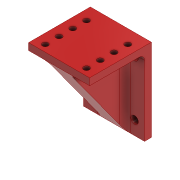
# Autodesk Inventor part: support
Saved by Autodesk Inventor 2020 (Build 240168000, 168)
## iProperties
Created: 2019-12-23
Part Number: support
Material: Generic
Document SubType Name: Modeling
Designer: ball
Density: 1 g/cm^3
Appearance: Default
Author: ball
Autodesk Inventor part; units mm, degrees
ref_plane "Work Plane1" through (172, 48, 15.3) normal (0, -1, 0) x (-1, 0, 0)
sketch "Sketch1" plane through (172, 48, 15.3) normal (0, -1, 0) x (-1, 0, 0)
  circle A0 centre (12, -16.7) radius 1.7 construction
  circle A1 centre (12, -32.7) radius 1.7 construction
  circle A2 centre (-12, 7.3) radius 1.7 construction
  circle A3 centre (-12, 15.3) radius 1.7 construction
  circle A4 centre (-12, 23.3) radius 1.7 construction
  circle A5 centre (-12, -24.7) radius 1.7 construction
  circle A6 centre (12, 23.3) radius 1.7 construction
  circle A7 centre (12, -56.7) radius 1.7 construction
  circle A8 centre (12, -48.7) radius 1.7 construction
  circle A9 centre (12, -40.7) radius 1.7 construction
  circle A10 centre (12, -8.7) radius 1.7 construction
  circle A11 centre (-12, -16.7) radius 1.7 construction
  circle A12 centre (12, -24.7) radius 1.7 construction
  circle A13 centre (-12, -0.7) radius 1.7 construction
  circle A14 centre (-12, -40.7) radius 1.7 construction
  circle A15 centre (-12, -48.7) radius 1.7 construction
  circle A16 centre (-12, -56.7) radius 1.7 construction
  circle A17 centre (-12, -32.7) radius 1.7 construction
  circle A18 centre (12, -80.7) radius 1.7 construction
  circle A19 centre (12, 15.3) radius 1.7 construction
  circle A20 centre (12, 7.3) radius 1.7 construction
  circle A21 centre (12, -0.7) radius 1.7 construction
  circle A22 centre (-12, -8.7) radius 1.7 construction
  circle A23 centre (-12, -80.7) radius 1.7 construction
  line L0 (10.05, 51.5627) -> (14.45, 51.5627) construction
  line L1 (14.45, 51.5627) -> (14.45, 45.5871) construction
  line L2 (14.45, 45.5871) -> (10.05, 45.5871) construction
  line L3 (10.05, 45.5871) -> (10.05, 51.5627) construction
  line L4 (10.05, -66.0122) -> (14.45, -66.0122) construction
  line L5 (14.45, -66.0122) -> (14.45, -71.9878) construction
  line L6 (14.45, -71.9878) -> (10.05, -71.9878) construction
  line L7 (10.05, -71.9878) -> (10.05, -66.0122) construction
  line L8 (-10.05, 75.3622) -> (-14.45, 75.3622) construction
  line L9 (-14.45, 75.3622) -> (-14.45, 81.3378) construction
  line L10 (-14.45, 81.3378) -> (-10.05, 81.3378) construction
  line L11 (-10.05, 81.3378) -> (-10.05, 75.3622) construction
  line L12 (-14.45, 56.302) -> (-10.05, 56.302) construction
  line L13 (-10.05, 56.302) -> (-10.05, 50.3264) construction
  line L14 (-10.05, 50.3264) -> (-14.45, 50.3264) construction
  line L15 (-14.45, 50.3264) -> (-14.45, 56.302) construction
  line L16 (9.5604, 33.925) -> (12.375, 35.55) construction
  line L17 (12.375, 35.55) -> (15.1896, 33.925) construction
  line L18 (15.1896, 33.925) -> (15.1896, 30.675) construction
  line L19 (15.1896, 30.675) -> (12.375, 29.05) construction
  line L20 (12.375, 29.05) -> (9.5604, 30.675) construction
  line L21 (9.5604, 30.675) -> (9.5604, 33.925) construction
  line L22 (2.8106, 33.925) -> (5.6252, 35.55) construction
  line L23 (5.6252, 35.55) -> (8.4398, 33.925) construction
  line L24 (8.4398, 33.925) -> (8.4398, 30.675) construction
  line L25 (8.4398, 30.675) -> (5.6252, 29.05) construction
  line L26 (5.6252, 29.05) -> (2.8106, 30.675) construction
  line L27 (2.8106, 30.675) -> (2.8106, 33.925) construction
  line L28 (3.2502, 68.3) -> (3.2502, 81) construction
  line L29 (3.2502, 81) -> (8.0002, 81) construction
  line L30 (8.0002, 81) -> (8.0002, 68.3) construction
  line L31 (8.0002, 68.3) -> (3.2502, 68.3) construction
  circle A24 centre (12.375, 40.3) radius 1.7 construction
  circle A25 centre (5.6252, 40.3) radius 1.7 construction
  line L32 (10.0002, 81) -> (14.75, 81) construction
  line L33 (14.75, 81) -> (14.75, 68.3) construction
  line L34 (14.75, 68.3) -> (10.0002, 68.3) construction
  line L35 (10.0002, 68.3) -> (10.0002, 81) construction
  line L36 (3.2502, 53.6) -> (3.2502, 66.3) construction
  line L37 (3.2502, 66.3) -> (8.0002, 66.3) construction
  line L38 (8.0002, 66.3) -> (8.0002, 53.6) construction
  line L39 (8.0002, 53.6) -> (3.2502, 53.6) construction
  circle A26 centre (-7.75, 60) radius 1.7 construction
  circle A27 centre (-7.75, -75) radius 1.7 construction
  line L40 (-6.125, 72.8146) -> (-4.5, 70) construction
  line L41 (-4.5, 70) -> (-6.125, 67.1854) construction
  line L42 (-6.125, 67.1854) -> (-9.375, 67.1854) construction
  line L43 (-9.375, 67.1854) -> (-11, 70) construction
  line L44 (-11, 70) -> (-9.375, 72.8146) construction
  line L45 (-9.375, 72.8146) -> (-6.125, 72.8146) construction
  line L46 (-6.125, -62.1854) -> (-4.5, -65) construction
  line L47 (-4.5, -65) -> (-6.125, -67.8146) construction
  line L48 (-6.125, -67.8146) -> (-9.375, -67.8146) construction
  line L49 (-9.375, -67.8146) -> (-11, -65) construction
  line L50 (-11, -65) -> (-9.375, -62.1854) construction
  line L51 (-9.375, -62.1854) -> (-6.125, -62.1854) construction
  line L52 (17.75, 85) -> (-17.75, 85) construction
  line L53 (-17.75, 85) -> (-17.75, -85) construction
  line L54 (-17.75, -85) -> (17.75, -85) construction
  line L55 (17.75, -85) -> (17.75, 85) construction
  line L56 (172, 15.3) -> (-20, 15.3) construction
  line L57 (-17.75, 15.3) -> (17.75, 15.3)
  line L58 (17.75, 15.3) -> (17.75, -20.6375)
  line L59 (17.75, -20.6375) -> (-17.75, -20.6375)
  line L60 (-17.75, 15.3) -> (-17.75, -20.6375)
  circle A28 centre (-12, 7.3) radius 1.7
  circle A29 centre (-12, -0.7) radius 1.7
  circle A30 centre (-12, -8.7) radius 1.7
  circle A31 centre (-12, -16.7) radius 1.7
  circle A32 centre (12, -16.7) radius 1.7
  circle A33 centre (12, -8.7) radius 1.7
  circle A34 centre (12, -0.7) radius 1.7
  circle A35 centre (12, 7.3) radius 1.7
  constraints: 8 centre point, 8 coincident, 8 concentric, 8 end point, 6 point on line, 2 perpendicular
extrude "Extrusion1" add sketch "Sketch1" along normal blind 4
ref_plane "Work Plane2" through (0, 0, 0) normal (0, 0, 1) x (1, 0, 0)
sketch "Sketch2" plane through (0, 0, 0) normal (0, 0, 1) x (1, 0, 0)
  line L0 (192, 0) -> (192, 48) construction
  line L1 (0, 48) -> (192, 48) construction
  line L2 (0, 0) -> (0, 48) construction
  line L3 (0, 0) -> (192, 0) construction
  circle A0 centre (168, 24) radius 7 construction
  circle A1 centre (144, 24) radius 7 construction
  arc A2 (160.9289, 33.8995) -> (158.1005, 31.0711) centre (159.5147, 32.4853) ccw construction
  line L4 (161.4142, 33.4142) -> (160.9289, 33.8995) construction
  arc A3 (158.5858, 30.5858) -> (161.4142, 33.4142) centre (160, 32) ccw construction
  line L5 (158.1005, 31.0711) -> (158.5858, 30.5858) construction
  line L6 (156.6863, 26) -> (155.3137, 26) construction
  arc A4 (156.6863, 22) -> (156.6863, 26) centre (156.6863, 24) ccw construction
  line L7 (155.3137, 22) -> (156.6863, 22) construction
  arc A5 (155.3137, 26) -> (155.3137, 22) centre (155.3137, 24) ccw construction
  arc A6 (158.1005, 16.9289) -> (160.9289, 14.1005) centre (159.5147, 15.5147) ccw construction
  line L8 (158.5858, 17.4142) -> (158.1005, 16.9289) construction
  arc A7 (161.4142, 14.5858) -> (158.5858, 17.4142) centre (160, 16) ccw construction
  line L9 (160.9289, 14.1005) -> (161.4142, 14.5858) construction
  arc A8 (177.8995, 31.0711) -> (175.0711, 33.8995) centre (176.4853, 32.4853) ccw construction
  line L10 (177.4142, 30.5858) -> (177.8995, 31.0711) construction
  arc A9 (174.5858, 33.4142) -> (177.4142, 30.5858) centre (176, 32) ccw construction
  line L11 (175.0711, 33.8995) -> (174.5858, 33.4142) construction
  arc A10 (180.6863, 22) -> (180.6863, 26) centre (180.6863, 24) ccw construction
  line L12 (179.3137, 22) -> (180.6863, 22) construction
  arc A11 (179.3137, 26) -> (179.3137, 22) centre (179.3137, 24) ccw construction
  line L13 (180.6863, 26) -> (179.3137, 26) construction
  line L14 (170, 35.3137) -> (170, 40) construction
  arc A12 (166, 35.3137) -> (170, 35.3137) centre (168, 35.3137) ccw construction
  line L15 (166, 40) -> (166, 35.3137) construction
  arc A13 (170, 40) -> (166, 40) centre (168, 40) ccw construction
  circle A14 centre (160, 40) radius 2 construction
  circle A15 centre (152, 40) radius 2 construction
  line L16 (146, 35.3137) -> (146, 40) construction
  arc A16 (142, 35.3137) -> (146, 35.3137) centre (144, 35.3137) ccw construction
  line L17 (142, 40) -> (142, 35.3137) construction
  arc A17 (146, 40) -> (142, 40) centre (144, 40) ccw construction
  circle A18 centre (136, 40) radius 2 construction
  circle A19 centre (128, 40) radius 2 construction
  line L18 (122, 35.3137) -> (122, 40) construction
  arc A20 (118, 35.3137) -> (122, 35.3137) centre (120, 35.3137) ccw construction
  line L19 (118, 40) -> (118, 35.3137) construction
  arc A21 (122, 40) -> (118, 40) centre (120, 40) ccw construction
  circle A22 centre (112, 40) radius 2 construction
  circle A23 centre (104, 40) radius 2 construction
  line L20 (98, 35.3137) -> (98, 40) construction
  arc A24 (94, 35.3137) -> (98, 35.3137) centre (96, 35.3137) ccw construction
  line L21 (94, 40) -> (94, 35.3137) construction
  arc A25 (98, 40) -> (94, 40) centre (96, 40) ccw construction
  circle A26 centre (88, 40) radius 2 construction
  circle A27 centre (80, 40) radius 2 construction
  line L22 (74, 35.3137) -> (74, 40) construction
  arc A28 (70, 35.3137) -> (74, 35.3137) centre (72, 35.3137) ccw construction
  line L23 (70, 40) -> (70, 35.3137) construction
  arc A29 (74, 40) -> (70, 40) centre (72, 40) ccw construction
  circle A30 centre (64, 40) radius 2 construction
  circle A31 centre (56, 40) radius 2 construction
  line L24 (50, 35.3137) -> (50, 40) construction
  arc A32 (46, 35.3137) -> (50, 35.3137) centre (48, 35.3137) ccw construction
  line L25 (46, 40) -> (46, 35.3137) construction
  arc A33 (50, 40) -> (46, 40) centre (48, 40) ccw construction
  circle A34 centre (40, 40) radius 2 construction
  circle A35 centre (32, 40) radius 2 construction
  line L26 (26, 35.3137) -> (26, 40) construction
  arc A36 (22, 35.3137) -> (26, 35.3137) centre (24, 35.3137) ccw construction
  line L27 (22, 40) -> (22, 35.3137) construction
  arc A37 (26, 40) -> (22, 40) centre (24, 40) ccw construction
  circle A38 centre (16, 40) radius 2 construction
  circle A39 centre (8, 40) radius 2 construction
  line L28 (166, 12.6863) -> (166, 8) construction
  arc A40 (170, 12.6863) -> (166, 12.6863) centre (168, 12.6863) ccw construction
  line L29 (170, 8) -> (170, 12.6863) construction
  arc A41 (166, 8) -> (170, 8) centre (168, 8) ccw construction
  circle A42 centre (160, 8) radius 2 construction
  circle A43 centre (152, 8) radius 2 construction
  line L30 (142, 12.6863) -> (142, 8) construction
  arc A44 (146, 12.6863) -> (142, 12.6863) centre (144, 12.6863) ccw construction
  line L31 (146, 8) -> (146, 12.6863) construction
  arc A45 (142, 8) -> (146, 8) centre (144, 8) ccw construction
  circle A46 centre (136, 8) radius 2 construction
  circle A47 centre (128, 8) radius 2 construction
  line L32 (118, 12.6863) -> (118, 8) construction
  arc A48 (122, 12.6863) -> (118, 12.6863) centre (120, 12.6863) ccw construction
  line L33 (122, 8) -> (122, 12.6863) construction
  arc A49 (118, 8) -> (122, 8) centre (120, 8) ccw construction
  circle A50 centre (112, 8) radius 2 construction
  circle A51 centre (104, 8) radius 2 construction
  line L34 (94, 12.6863) -> (94, 8) construction
  arc A52 (98, 12.6863) -> (94, 12.6863) centre (96, 12.6863) ccw construction
  line L35 (98, 8) -> (98, 12.6863) construction
  arc A53 (94, 8) -> (98, 8) centre (96, 8) ccw construction
  circle A54 centre (88, 8) radius 2 construction
  circle A55 centre (80, 8) radius 2 construction
  line L36 (70, 12.6863) -> (70, 8) construction
  arc A56 (74, 12.6863) -> (70, 12.6863) centre (72, 12.6863) ccw construction
  line L37 (74, 8) -> (74, 12.6863) construction
  arc A57 (70, 8) -> (74, 8) centre (72, 8) ccw construction
  circle A58 centre (64, 8) radius 2 construction
  circle A59 centre (56, 8) radius 2 construction
  line L38 (46, 12.6863) -> (46, 8) construction
  arc A60 (50, 12.6863) -> (46, 12.6863) centre (48, 12.6863) ccw construction
  line L39 (50, 8) -> (50, 12.6863) construction
  arc A61 (46, 8) -> (50, 8) centre (48, 8) ccw construction
  circle A62 centre (40, 8) radius 2 construction
  circle A63 centre (32, 8) radius 2 construction
  line L40 (22, 12.6863) -> (22, 8) construction
  arc A64 (26, 12.6863) -> (22, 12.6863) centre (24, 12.6863) ccw construction
  line L41 (26, 8) -> (26, 12.6863) construction
  arc A65 (22, 8) -> (26, 8) centre (24, 8) ccw construction
  circle A66 centre (16, 8) radius 2 construction
  circle A67 centre (8, 8) radius 2 construction
  arc A68 (9.8995, 31.0711) -> (7.0711, 33.8995) centre (8.4853, 32.4853) ccw construction
  line L42 (9.4142, 30.5858) -> (9.8995, 31.0711) construction
  arc A69 (6.5858, 33.4142) -> (9.4142, 30.5858) centre (8, 32) ccw construction
  line L43 (7.0711, 33.8995) -> (6.5858, 33.4142) construction
  arc A70 (7.0711, 14.1005) -> (9.8995, 16.9289) centre (8.4853, 15.5147) ccw construction
  line L44 (6.5858, 14.5858) -> (7.0711, 14.1005) construction
  arc A71 (9.4142, 17.4142) -> (6.5858, 14.5858) centre (8, 16) ccw construction
  line L45 (9.8995, 16.9289) -> (9.4142, 17.4142) construction
  arc A72 (184.9289, 33.8995) -> (182.1005, 31.0711) centre (183.5147, 32.4853) ccw construction
  line L46 (185.4142, 33.4142) -> (184.9289, 33.8995) construction
  arc A73 (182.5858, 30.5858) -> (185.4142, 33.4142) centre (184, 32) ccw construction
  line L47 (182.1005, 31.0711) -> (182.5858, 30.5858) construction
  arc A74 (182.1005, 16.9289) -> (184.9289, 14.1005) centre (183.5147, 15.5147) ccw construction
  line L48 (182.5858, 17.4142) -> (182.1005, 16.9289) construction
  arc A75 (185.4142, 14.5858) -> (182.5858, 17.4142) centre (184, 16) ccw construction
  line L49 (184.9289, 14.1005) -> (185.4142, 14.5858) construction
  circle A76 centre (176, 8) radius 2 construction
  circle A77 centre (176, 40) radius 2 construction
  circle A78 centre (184, 40) radius 2 construction
  circle A79 centre (184, 8) radius 2 construction
  arc A80 (33.8995, 31.0711) -> (31.0711, 33.8995) centre (32.4853, 32.4853) ccw construction
  line L50 (33.4142, 30.5858) -> (33.8995, 31.0711) construction
  arc A81 (30.5858, 33.4142) -> (33.4142, 30.5858) centre (32, 32) ccw construction
  line L51 (31.0711, 33.8995) -> (30.5858, 33.4142) construction
  arc A82 (57.8995, 31.0711) -> (55.0711, 33.8995) centre (56.4853, 32.4853) ccw construction
  line L52 (57.4142, 30.5858) -> (57.8995, 31.0711) construction
  arc A83 (54.5858, 33.4142) -> (57.4142, 30.5858) centre (56, 32) ccw construction
  line L53 (55.0711, 33.8995) -> (54.5858, 33.4142) construction
  arc A84 (81.8995, 31.0711) -> (79.0711, 33.8995) centre (80.4853, 32.4853) ccw construction
  line L54 (81.4142, 30.5858) -> (81.8995, 31.0711) construction
  arc A85 (78.5858, 33.4142) -> (81.4142, 30.5858) centre (80, 32) ccw construction
  line L55 (79.0711, 33.8995) -> (78.5858, 33.4142) construction
  arc A86 (105.8995, 31.0711) -> (103.0711, 33.8995) centre (104.4853, 32.4853) ccw construction
  line L56 (105.4142, 30.5858) -> (105.8995, 31.0711) construction
  arc A87 (102.5858, 33.4142) -> (105.4142, 30.5858) centre (104, 32) ccw construction
  line L57 (103.0711, 33.8995) -> (102.5858, 33.4142) construction
  arc A88 (129.8995, 31.0711) -> (127.0711, 33.8995) centre (128.4853, 32.4853) ccw construction
  line L58 (129.4142, 30.5858) -> (129.8995, 31.0711) construction
  arc A89 (126.5858, 33.4142) -> (129.4142, 30.5858) centre (128, 32) ccw construction
  line L59 (127.0711, 33.8995) -> (126.5858, 33.4142) construction
  arc A90 (153.8995, 31.0711) -> (151.0711, 33.8995) centre (152.4853, 32.4853) ccw construction
  line L60 (153.4142, 30.5858) -> (153.8995, 31.0711) construction
  arc A91 (150.5858, 33.4142) -> (153.4142, 30.5858) centre (152, 32) ccw construction
  line L61 (151.0711, 33.8995) -> (150.5858, 33.4142) construction
  arc A92 (14.1005, 16.9289) -> (16.9289, 14.1005) centre (15.5147, 15.5147) ccw construction
  line L62 (14.5858, 17.4142) -> (14.1005, 16.9289) construction
  arc A93 (17.4142, 14.5858) -> (14.5858, 17.4142) centre (16, 16) ccw construction
  line L63 (16.9289, 14.1005) -> (17.4142, 14.5858) construction
  arc A94 (38.1005, 16.9289) -> (40.9289, 14.1005) centre (39.5147, 15.5147) ccw construction
  line L64 (38.5858, 17.4142) -> (38.1005, 16.9289) construction
  arc A95 (41.4142, 14.5858) -> (38.5858, 17.4142) centre (40, 16) ccw construction
  line L65 (40.9289, 14.1005) -> (41.4142, 14.5858) construction
  arc A96 (62.1005, 16.9289) -> (64.9289, 14.1005) centre (63.5147, 15.5147) ccw construction
  line L66 (62.5858, 17.4142) -> (62.1005, 16.9289) construction
  arc A97 (65.4142, 14.5858) -> (62.5858, 17.4142) centre (64, 16) ccw construction
  line L67 (64.9289, 14.1005) -> (65.4142, 14.5858) construction
  arc A98 (86.1005, 16.9289) -> (88.9289, 14.1005) centre (87.5147, 15.5147) ccw construction
  line L68 (86.5858, 17.4142) -> (86.1005, 16.9289) construction
  arc A99 (89.4142, 14.5858) -> (86.5858, 17.4142) centre (88, 16) ccw construction
  line L69 (88.9289, 14.1005) -> (89.4142, 14.5858) construction
  arc A100 (110.1005, 16.9289) -> (112.9289, 14.1005) centre (111.5147, 15.5147) ccw construction
  line L70 (110.5858, 17.4142) -> (110.1005, 16.9289) construction
  arc A101 (113.4142, 14.5858) -> (110.5858, 17.4142) centre (112, 16) ccw construction
  line L71 (112.9289, 14.1005) -> (113.4142, 14.5858) construction
  arc A102 (134.1005, 16.9289) -> (136.9289, 14.1005) centre (135.5147, 15.5147) ccw construction
  line L72 (134.5858, 17.4142) -> (134.1005, 16.9289) construction
  arc A103 (137.4142, 14.5858) -> (134.5858, 17.4142) centre (136, 16) ccw construction
  line L73 (136.9289, 14.1005) -> (137.4142, 14.5858) construction
  line L74 (11.3137, 22) -> (12.6863, 22) construction
  arc A104 (11.3137, 26) -> (11.3137, 22) centre (11.3137, 24) ccw construction
  line L75 (12.6863, 26) -> (11.3137, 26) construction
  arc A105 (12.6863, 22) -> (12.6863, 26) centre (12.6863, 24) ccw construction
  line L76 (36.6863, 26) -> (35.3137, 26) construction
  arc A106 (36.6863, 22) -> (36.6863, 26) centre (36.6863, 24) ccw construction
  line L77 (35.3137, 22) -> (36.6863, 22) construction
  arc A107 (35.3137, 26) -> (35.3137, 22) centre (35.3137, 24) ccw construction
  line L78 (60.6863, 26) -> (59.3137, 26) construction
  arc A108 (60.6863, 22) -> (60.6863, 26) centre (60.6863, 24) ccw construction
  line L79 (59.3137, 22) -> (60.6863, 22) construction
  arc A109 (59.3137, 26) -> (59.3137, 22) centre (59.3137, 24) ccw construction
  line L80 (84.6863, 26) -> (83.3137, 26) construction
  arc A110 (84.6863, 22) -> (84.6863, 26) centre (84.6863, 24) ccw construction
  line L81 (83.3137, 22) -> (84.6863, 22) construction
  arc A111 (83.3137, 26) -> (83.3137, 22) centre (83.3137, 24) ccw construction
  line L82 (108.6863, 26) -> (107.3137, 26) construction
  arc A112 (108.6863, 22) -> (108.6863, 26) centre (108.6863, 24) ccw construction
  line L83 (107.3137, 22) -> (108.6863, 22) construction
  arc A113 (107.3137, 26) -> (107.3137, 22) centre (107.3137, 24) ccw construction
  line L84 (132.6863, 26) -> (131.3137, 26) construction
  arc A114 (132.6863, 22) -> (132.6863, 26) centre (132.6863, 24) ccw construction
  line L85 (131.3137, 22) -> (132.6863, 22) construction
  arc A115 (131.3137, 26) -> (131.3137, 22) centre (131.3137, 24) ccw construction
  arc A116 (16.9289, 33.8995) -> (14.1005, 31.0711) centre (15.5147, 32.4853) ccw construction
  line L86 (17.4142, 33.4142) -> (16.9289, 33.8995) construction
  arc A117 (14.5858, 30.5858) -> (17.4142, 33.4142) centre (16, 32) ccw construction
  line L87 (14.1005, 31.0711) -> (14.5858, 30.5858) construction
  arc A118 (40.9289, 33.8995) -> (38.1005, 31.0711) centre (39.5147, 32.4853) ccw construction
  line L88 (41.4142, 33.4142) -> (40.9289, 33.8995) construction
  arc A119 (38.5858, 30.5858) -> (41.4142, 33.4142) centre (40, 32) ccw construction
  line L89 (38.1005, 31.0711) -> (38.5858, 30.5858) construction
  arc A120 (64.9289, 33.8995) -> (62.1005, 31.0711) centre (63.5147, 32.4853) ccw construction
  line L90 (65.4142, 33.4142) -> (64.9289, 33.8995) construction
  arc A121 (62.5858, 30.5858) -> (65.4142, 33.4142) centre (64, 32) ccw construction
  line L91 (62.1005, 31.0711) -> (62.5858, 30.5858) construction
  arc A122 (88.9289, 33.8995) -> (86.1005, 31.0711) centre (87.5147, 32.4853) ccw construction
  line L92 (89.4142, 33.4142) -> (88.9289, 33.8995) construction
  arc A123 (86.5858, 30.5858) -> (89.4142, 33.4142) centre (88, 32) ccw construction
  line L93 (86.1005, 31.0711) -> (86.5858, 30.5858) construction
  arc A124 (112.9289, 33.8995) -> (110.1005, 31.0711) centre (111.5147, 32.4853) ccw construction
  line L94 (113.4142, 33.4142) -> (112.9289, 33.8995) construction
  arc A125 (110.5858, 30.5858) -> (113.4142, 33.4142) centre (112, 32) ccw construction
  line L95 (110.1005, 31.0711) -> (110.5858, 30.5858) construction
  arc A126 (136.9289, 33.8995) -> (134.1005, 31.0711) centre (135.5147, 32.4853) ccw construction
  line L96 (137.4142, 33.4142) -> (136.9289, 33.8995) construction
  arc A127 (134.5858, 30.5858) -> (137.4142, 33.4142) centre (136, 32) ccw construction
  line L97 (134.1005, 31.0711) -> (134.5858, 30.5858) construction
  arc A128 (31.0711, 14.1005) -> (33.8995, 16.9289) centre (32.4853, 15.5147) ccw construction
  line L98 (30.5858, 14.5858) -> (31.0711, 14.1005) construction
  arc A129 (33.4142, 17.4142) -> (30.5858, 14.5858) centre (32, 16) ccw construction
  line L99 (33.8995, 16.9289) -> (33.4142, 17.4142) construction
  arc A130 (55.0711, 14.1005) -> (57.8995, 16.9289) centre (56.4853, 15.5147) ccw construction
  line L100 (54.5858, 14.5858) -> (55.0711, 14.1005) construction
  arc A131 (57.4142, 17.4142) -> (54.5858, 14.5858) centre (56, 16) ccw construction
  line L101 (57.8995, 16.9289) -> (57.4142, 17.4142) construction
  arc A132 (79.0711, 14.1005) -> (81.8995, 16.9289) centre (80.4853, 15.5147) ccw construction
  line L102 (78.5858, 14.5858) -> (79.0711, 14.1005) construction
  arc A133 (81.4142, 17.4142) -> (78.5858, 14.5858) centre (80, 16) ccw construction
  line L103 (81.8995, 16.9289) -> (81.4142, 17.4142) construction
  arc A134 (103.0711, 14.1005) -> (105.8995, 16.9289) centre (104.4853, 15.5147) ccw construction
  line L104 (102.5858, 14.5858) -> (103.0711, 14.1005) construction
  arc A135 (105.4142, 17.4142) -> (102.5858, 14.5858) centre (104, 16) ccw construction
  line L105 (105.8995, 16.9289) -> (105.4142, 17.4142) construction
  arc A136 (127.0711, 14.1005) -> (129.8995, 16.9289) centre (128.4853, 15.5147) ccw construction
  line L106 (126.5858, 14.5858) -> (127.0711, 14.1005) construction
  arc A137 (129.4142, 17.4142) -> (126.5858, 14.5858) centre (128, 16) ccw construction
  line L107 (129.8995, 16.9289) -> (129.4142, 17.4142) construction
  arc A138 (151.0711, 14.1005) -> (153.8995, 16.9289) centre (152.4853, 15.5147) ccw construction
  line L108 (150.5858, 14.5858) -> (151.0711, 14.1005) construction
  arc A139 (153.4142, 17.4142) -> (150.5858, 14.5858) centre (152, 16) ccw construction
  line L109 (153.8995, 16.9289) -> (153.4142, 17.4142) construction
  arc A140 (175.0711, 14.1005) -> (177.8995, 16.9289) centre (176.4853, 15.5147) ccw construction
  line L110 (174.5858, 14.5858) -> (175.0711, 14.1005) construction
  arc A141 (177.4142, 17.4142) -> (174.5858, 14.5858) centre (176, 16) ccw construction
  line L111 (177.8995, 16.9289) -> (177.4142, 17.4142) construction
  circle A142 centre (24, 24) radius 7 construction
  circle A143 centre (48, 24) radius 7 construction
  circle A144 centre (72, 24) radius 7 construction
  circle A145 centre (96, 24) radius 7 construction
  circle A146 centre (120, 24) radius 7 construction
  circle A147 centre (184, 8) radius 2.2
  circle A148 centre (184, 40) radius 2.2
  circle A149 centre (160, 40) radius 2.2
  circle A150 centre (160, 8) radius 2.2
  line L112 (154.25, 44) -> (189.75, 44) projected
  line L113 (154.25, 44) -> (154.25, 0)
  line L114 (189.75, 0) -> (154.25, 0)
  line L115 (154.25, 44) -> (189.75, 44)
  line L116 (189.75, 48) -> (189.75, 44) projected
  line L117 (189.75, 44) -> (189.75, 0)
  point P0 (192, 44)
  dimension "d2" = 4.4
  dimension "d3" = 4.4
  dimension "d4" = 4.4
  dimension "d5" = 4.4
  constraints: 8 end point, 4 centre point, 4 coincident, 2 perpendicular, 2 point on line, 1 collinear, 1 parallel
  measures "d2" diameter of A147
  measures "d3" diameter of A148
  measures "d4" diameter of A149
  measures "d5" diameter of A150
extrude "Extrusion2" add sketch "Sketch2" along normal blind 4
ref_plane "Work Plane3" through (172, 48, 35.9375) normal (1, 0, 0) x (0, 0, -1)
sketch "Sketch3" plane through (172, 48, 35.9375) normal (1, 0, 0) x (0, 0, -1)
  line L0 (31.9375, -48) -> (31.9375, -4) projected
  line L1 (31.9375, -4) -> (0, -4) projected
  line L2 (31.9375, -48) -> (31.9375, -4)
  line L3 (0, -4) -> (31.9375, -48)
  point P0 (35.9375, -48)
  constraints: 5 end point
extrude "Extrusion3" add sketch "Sketch3" along normal mid plane 12.7
fillet "Fillet1" radius 3.175 4 edges at (178.35, 44, 19.9688) (178.35, 22, 4) (165.65, 22, 4) (165.65, 44, 19.9688)
fillet "Fillet2" radius 3.175 4 edges at (179.2799, 43.0701, 4.9299) (185.6375, 44, 4) (164.7201, 43.0701, 4.9299) (158.3625, 44, 4)
body "Solid1"
